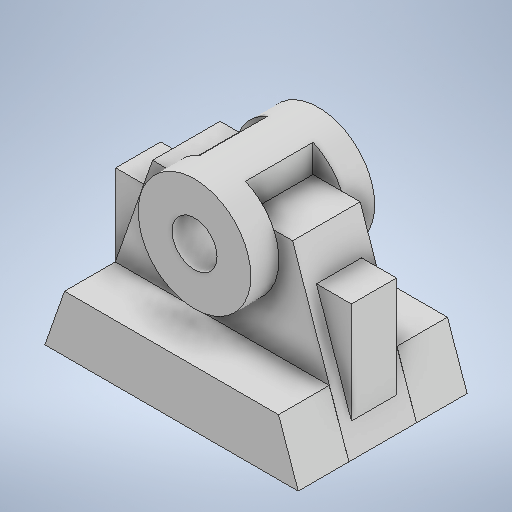
# Autodesk Inventor part: Q2 auto
Saved by Autodesk Inventor 2025.2 (Build 292293000, 293)
## iProperties
Created: 2025-03-19
Part Number: Q2 auto
Material: Generic
Document SubType Name: Modeling
Designer: rajan
Density: 1 g/cm^3
Appearance: Default
Author: rajan
Autodesk Inventor part; units mm, degrees
ref_plane "YZ Plane" through (0, 0, 0) normal (1, 0, 0) x (0, 1, 0)
ref_plane "XZ Plane" through (0, 0, 0) normal (0, 1, 0) x (-1, 0, 0)
ref_plane "XY Plane" through (0, 0, 0) normal (0, 0, 1) x (1, 0, 0)
sketch "Sketch1" plane through (0, 0, 0) normal (0, 0, 1) x (1, 0, 0)
  line L0 (-45, 0) -> (45, 0)
  circle A0 centre (0.1619, 49.6388) radius 8
  circle A1 centre (0.1619, 49.6388) radius 20
  line L1 (-7.7534, 57.876) -> (-7.7534, 68.0058)
  line L2 (-7.7534, 57.876) -> (-18.063, 57.876)
  line L3 (8.2464, 58) -> (18.3303, 58)
  line L4 (8.2464, 58) -> (8.2464, 67.932)
  line L5 (25, 58) -> (18.3303, 58)
  line L6 (-24.7326, 57.9068) -> (-18.063, 57.876)
  line L7 (45, 0) -> (-45, 0)
  line L8 (-41.85, 9) -> (-41.85, 45)
  line L9 (-41.85, 45) -> (-29.25, 45)
  line L10 (41.8966, 9) -> (41.8966, 45)
  line L11 (41.8966, 45) -> (29.4828, 45)
  line L12 (-38, 20) -> (38, 20)
  line L13 (-45, 0) -> (-24.7326, 57.9068)
  line L14 (25, 58) -> (45, 0)
  line L15 (-45, 0) -> (-38, 20)
  line L16 (38, 20) -> (45, 0)
  point P0 (0, 0)
  constraints: 34 end point, 5 horizontal, 4 point on circle, 4 vertical, 2 centre point, 2 perpendicular, 1 coincident, 1 collinear
extrude "Extrusion1" add sketch "Sketch1" along normal mid plane 44 contours A1 L2 L1 L4 L3
extrude "Extrusion2" add sketch "Sketch1" along normal mid plane 44 contours L3 L4 A1
extrude "Extrusion3" add sketch "Sketch1" along normal mid plane 44 contours A1 L1 L2
extrude "Extrusion4" cut sketch "Sketch1" along normal mid plane 24 contours A1 L1 L2
extrude "Extrusion5" cut sketch "Sketch1" along normal mid plane 24 contours L3 L4 A1
extrude "Extrusion6" add sketch "Sketch1" along normal mid plane 16 contours L14 L11 L10
extrude "Extrusion7" add sketch "Sketch1" along normal mid plane 16 contours L8 L9 L13
extrude "Extrusion8" add sketch "Sketch1" along normal mid plane 24 contours L16 L12 L13 L6 A1 L5 L14
extrude "Extrusion9" add sketch "Sketch1" along normal mid plane 60 contours L13 L12 L16 L0
body "Solid1"
